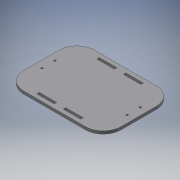
# Autodesk Inventor part: base_plate
Saved by Autodesk Inventor 2017 (Build 210142000, 142)
## iProperties
Created: 2017-06-15
Part Number: base_plate
Material: Generic
Document SubType Name: Modeling
Designer: millerid
Density: 1 g/cm^3
Appearance: Default
Author: millerid
Autodesk Inventor part; units mm, degrees
ref_plane "YZ Plane" through (0, 0, 0) normal (1, 0, 0) x (0, 1, 0)
ref_plane "XZ Plane" through (0, 0, 0) normal (0, 1, 0) x (-1, 0, 0)
ref_plane "XY Plane" through (0, 0, 0) normal (0, 0, 1) x (1, 0, 0)
sketch "Sketch1" plane through (0, 0, 0) normal (0, 1, 0) x (-1, 0, 0)
  line L0 (20, 0) -> (89.97, 0)
  line L1 (109.97, -20) -> (109.97, -60)
  line L2 (89.97, -80) -> (20, -80)
  line L3 (0, -60) -> (0, -20)
  line L4 (79.7968, -72.5282) -> (60, -72.5282)
  line L5 (60, -72.5282) -> (60, -75.5)
  line L6 (60, -75.5) -> (79.7968, -75.5)
  line L7 (79.7968, -75.5) -> (79.7968, -72.5282)
  circle A0 centre (101.97, -32.634) radius 1.143
  circle A1 centre (101.97, -47.366) radius 1.143
  circle A2 centre (8, -35.134) radius 1.143
  circle A3 centre (8, -49.866) radius 1.143
  arc A4 (109.97, -20) -> (89.97, 0) centre (89.97, -20) ccw
  arc A5 (0, -60) -> (20, -80) centre (20, -60) ccw
  arc A6 (89.97, -80) -> (109.97, -60) centre (89.97, -60) ccw
  arc A7 (20, 0) -> (0, -20) centre (20, -20) ccw
  line L8 (49.7968, -4.5282) -> (30, -4.5282)
  line L9 (30, -4.5282) -> (30, -7.5)
  line L10 (30, -7.5) -> (49.7968, -7.5)
  line L11 (49.7968, -7.5) -> (49.7968, -4.5282)
  line L12 (49.7968, -72.5282) -> (30, -72.5282)
  line L13 (30, -72.5282) -> (30, -75.5)
  line L14 (30, -75.5) -> (49.7968, -75.5)
  line L15 (49.7968, -75.5) -> (49.7968, -72.5282)
  line L16 (60, -7.5) -> (79.7968, -7.5)
  line L17 (79.7968, -7.5) -> (79.7968, -4.5282)
  line L18 (79.7968, -4.5282) -> (60, -4.5282)
  line L19 (60, -4.5282) -> (60, -7.5)
  point P0 (0, 0)
  point P1 (109.97, -80)
  point P2 (109.97, 0)
  point P3 (0, -80)
  dimension "d0" = 109.97
  dimension "d1" = 80
  dimension "d2" = 19.7968
  dimension "d3" = 2.9718
  dimension "d7" = 4.5
  dimension "d9" = 2.286
  dimension "d10" = 2.286
  dimension "d11" = 14.732
  dimension "d12" = 32.634
  dimension "d13" = 8
  dimension "d14" = 8
  dimension "d15" = 2.286
  dimension "d16" = 2.286
  dimension "d17" = 8
  dimension "d18" = 8
  dimension "d19" = 20
  dimension "d20" = 20
  dimension "d21" = 20
  dimension "d24" = 19.7968
  dimension "d25" = 30
  dimension "d30" = 2.9718
  constraints: 40 end point, 10 parallel, 8 centre point, 8 collinear, 8 point on circle, 8 point on line, 8 tangent, 5 horizontal, 5 perpendicular, 1 equal radius
  measures "d0" distance of point (109.97, -80) point (0, -80)
  measures "d1" distance of point (109.97, 0) point (109.97, -80)
  measures "d2" distance of L6.end L5.end
  measures "d3" distance of L5.end L4.end
  measures "d7" distance between parallel lines of L2 L6
  measures "d9" diameter of A0
  measures "d10" diameter of A1
  measures "d11" distance of A1.centre A0.centre
  measures "d12" distance from line of L0 A0.centre
  measures "d13" distance from line of L1 A1.centre
  measures "d14" distance from line of A0.centre L1
  measures "d15" diameter of A2
  measures "d16" diameter of A3
  measures "d17" distance from line of L3 A2.centre
  measures "d18" distance from line of L3 A3.centre
  measures "d19" radius of A4
  measures "d20" radius of A5
  measures "d21" radius of A7
  measures "d24" distance of L10.end L9.end
  measures "d25" distance between parallel lines of L9 L3
  measures "d30" distance between parallel lines of L8 L10
extrude "Extrusion4" add sketch "Sketch1" along normal blind 3.175
equation "\"d10\" = d9"
equation "\"d12\" = -0.5 * d11 + 0.5 * d1"
equation "\"d15\" = d9"
equation "\"d16\" = d9"
equation "\"d24\" = d2"
equation "\"d30\" = d3"
body "Solid4"
